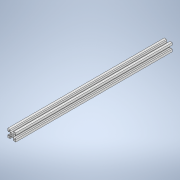
# Autodesk Inventor part: V-SLOT_2020
Saved by Autodesk Inventor 2021 (Build 250183000, 183)
## iProperties
Created: 2022-05-21
Part Number: V-SLOT_2020
Material: Aluminio
Document SubType Name: Modeling
Designer: 79449
Density: 2.7 g/cm^3
Appearance: Satinado
Author: 79449
Autodesk Inventor part; units mm, degrees
ref_plane "YZ Plane" through (0, 0, 0) normal (1, 0, 0) x (0, 1, 0)
ref_plane "XZ Plane" through (0, 0, 0) normal (0, 1, 0) x (-1, 0, 0)
ref_plane "XY Plane" through (0, 0, 0) normal (0, 0, 1) x (1, 0, 0)
sketch "Boceto1" plane through (0, 0, 0) normal (0, 0, 1) x (1, 0, 0)
  line L0 (30, 10) -> (30, -10) construction
  line L1 (20, -10) -> (20, 10) construction
  circle A0 centre (20, 0) radius 2.1
  line L2 (22.8393, 3.9) -> (17.1607, 3.9)
  line L3 (17.1607, -3.9) -> (22.8393, -3.9)
  line L4 (23.9, -2.8393) -> (23.9, 2.8393)
  line L5 (20, 10) -> (20, -10) construction
  line L6 (25.5, 6.5607) -> (25.5, 8.2)
  line L7 (23.9, 3.9) -> (25.9093, 5.9093) construction
  line L8 (26.5607, 5.5) -> (23.9, 2.8393)
  line L9 (22.8393, 3.9) -> (25.5, 6.5607)
  line L10 (24.58, 10) -> (22.78, 8.2)
  line L11 (27, -5.9393) -> (27, -8.2) construction
  line L12 (25.5, -6.5607) -> (25.5, -8.2)
  line L13 (26.5607, -5.5) -> (23.9, -2.8393)
  line L14 (23.9, -3.9) -> (25.9093, -5.9093) construction
  line L15 (22.8393, -3.9) -> (25.5, -6.5607)
  line L16 (24.58, -10) -> (22.78, -8.2)
  line L17 (22.78, -8.2) -> (25.5, -8.2)
  line L18 (27.1393, -8.2) -> (30, -8.2) construction
  line L19 (25.5, 8.2) -> (22.78, 8.2)
  line L20 (30, -10) -> (30, 10) construction
  line L21 (24.58, 10) -> (30, 10)
  line L22 (24.58, -10) -> (30, -10)
  line L23 (30, -10) -> (30, -8.2)
  line L24 (30, 8.2) -> (30, 10)
  line L25 (28.2, -10) -> (28.2, -5.5) construction
  line L26 (28.2, -5.5) -> (28.2, -2.7333)
  line L27 (25.5, -6.5607) -> (26.5607, -5.5) construction
  line L28 (26.5607, -5.5) -> (28.2, -5.5)
  line L29 (28.2, -2.7333) -> (30, -4.5333)
  line L30 (30, -8.2) -> (30, -4.5333)
  line L31 (26.5607, 5.5) -> (23.9, 2.8393)
  line L32 (30, 10) -> (30, 8.2)
  line L33 (28.2, 5.5) -> (28.2, 2.7333)
  line L34 (26.5607, 5.5) -> (28.2, 5.5)
  line L35 (28.2, 2.7333) -> (30, 4.5333)
  line L36 (30, 8.2) -> (30, 4.5333)
  line L37 (10, 10) -> (10, -10) construction
  line L38 (15.42, 10) -> (17.22, 8.2)
  line L39 (14.5, 8.2) -> (17.22, 8.2)
  line L40 (15.42, 10) -> (10, 10)
  line L41 (16.1, -2.8393) -> (16.1, 2.8393)
  line L42 (16.1, -3.9) -> (14.0907, -5.9093) construction
  line L43 (17.22, -8.2) -> (14.5, -8.2)
  line L44 (17.1607, 3.9) -> (22.8393, 3.9)
  circle A1 centre (20, 0) radius 2.1
  line L45 (22.8393, -3.9) -> (17.1607, -3.9)
  line L46 (15.42, -10) -> (17.22, -8.2)
  line L47 (14.5, -6.5607) -> (14.5, -8.2)
  line L48 (12.8607, -8.2) -> (10, -8.2) construction
  line L49 (15.42, -10) -> (10, -10)
  line L50 (14.5, 6.5607) -> (14.5, 8.2)
  line L51 (16.1, 3.9) -> (14.0907, 5.9093) construction
  line L52 (13.4393, 5.5) -> (16.1, 2.8393)
  line L53 (17.1607, 3.9) -> (14.5, 6.5607)
  line L54 (17.1607, -3.9) -> (14.5, -6.5607)
  line L55 (13.4393, -5.5) -> (16.1, -2.8393)
  line L56 (13, -5.9393) -> (13, -8.2) construction
  line L57 (10, -10) -> (10, 10) construction
  line L58 (10, -10) -> (10, -8.2)
  line L59 (10, 8.2) -> (10, 10)
  line L60 (11.8, -10) -> (11.8, -5.5) construction
  line L61 (11.8, -5.5) -> (11.8, -2.7333)
  line L62 (14.5, -6.5607) -> (13.4393, -5.5) construction
  line L63 (13.4393, -5.5) -> (11.8, -5.5)
  line L64 (11.8, -2.7333) -> (10, -4.5333)
  line L65 (10, -8.2) -> (10, -4.5333)
  line L66 (13.4393, 5.5) -> (16.1, 2.8393)
  line L67 (13.4393, 5.5) -> (11.8, 5.5)
  line L68 (11.8, 5.5) -> (11.8, 2.7333)
  line L69 (11.8, 2.7333) -> (10, 4.5333)
  line L70 (10, 8.2) -> (10, 4.5333)
  line L71 (10, 10) -> (10, 8.2)
  dimension "d9" = 20
  dimension "d53" = 10
  dimension "d56" = 1.6393
  dimension "d58" = 2.72
  dimension "d66" = 1.8
  dimension "d71" = 45
  dimension "d72" = 2.6607
  dimension "d77" = 4.2
  dimension "d78" = 3.9
  dimension "d79" = 3.9
  dimension "d80" = 3.9
  dimension "d81" = 1.5
  dimension "d82" = 45
  dimension "d83" = 90
  dimension "d84" = 45
  dimension "d85" = 5.42
  dimension "d86" = 1.5
  dimension "d87" = 90
  dimension "d88" = 5.42
  dimension "d89" = 5.4667
  dimension "d90" = 5.6787
  dimension "d91" = 5.6787
  dimension "d92" = 5.6787
  dimension "d93" = 2.6607
  dimension "d94" = 2.6607
  dimension "d95" = 2.6607
  constraints: 144 end point, 37 symmetric about line, 6 point on line, 3 collinear, 2 centre point, 1 horizontal, 1 perpendicular, 1 vertical, 1 other
  measures "d9" distance of L0.start L0.end
  measures "d53" distance between parallel lines of L0 L1
  measures "d56" distance of L12.start L17.end
  measures "d58" distance of L17.start L17.end
  measures "d66" distance between parallel lines of L25 L20
  measures "d71" angle of L26 L29
  measures "d72" horizontal distance of L13.start L4.start
  measures "d77" diameter of A0
  measures "d78" distance from line of A0.centre L2
  measures "d79" distance from line of L3 A0.centre
  measures "d80" distance from line of L4 point (20, 0)
  measures "d81" distance between parallel lines of L31 L9
  measures "d82" angle of L10 L32
  measures "d83" angle of L6 L34
  measures "d84" angle of L35 L33
  measures "d85" distance of L10.start L21.end
  measures "d86" distance between parallel lines of L15 L13
  measures "d87" angle of L12 L28
  measures "d88" distance of L16.start L22.end
  measures "d89" distance of L29.end L22.end
  measures "d90" distance of L4.start L4.end
  measures "d91" distance of L2.start L2.end
  measures "d92" distance of L3.start L3.end
  measures "d93" horizontal distance of L8.start L4.end
  measures "d94" horizontal distance of L2.start L6.start
  measures "d95" horizontal distance of L3.end L12.start
extrude "Extrusión1" add sketch "Boceto1" along normal blind 390
